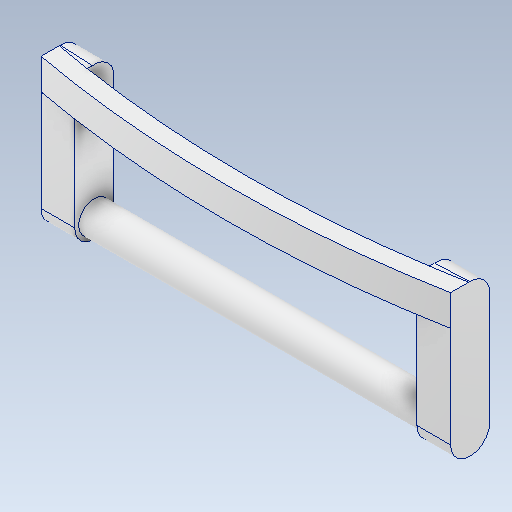
# Autodesk Inventor part: Watch Top strap attachment
Saved by Autodesk Inventor 2020 (Build 240168000, 168)
## iProperties
Created: 2020-05-09
Part Number: Watch Top strap attachment
Material: Aluminum 6061
Document SubType Name: Modeling
Designer: harry
Density: 2.7 g/cm^3
Appearance: Aluminum - Flat
Author: harry
Autodesk Inventor part; units mm, degrees
ref_plane "YZ Plane" through (0, 0, 0) normal (1, 0, 0) x (0, 1, 0)
ref_plane "XY Plane" through (0, 0, 0) normal (0, 0, 1) x (1, 0, 0)
sketch "Sketch1" plane through (0, 0, 0) normal (1, 0, 0) x (0, 1, 0)
  circle A0 centre (0, 0) radius 1.4
  dimension "d0" = 2.8
  constraints: 1 centre point, 1 coincident
  measures "d0" diameter of A0
extrude "Extrusion1" add sketch "Sketch1" along normal mid plane 30.5
sketch "Sketch2" plane through (15.25, 0, 0) normal (1, 0, 0) x (0, 0, -1)
  arc A0 (-1.75, 0) -> (1.75, 0) centre (0, 0) ccw
  line L0 (-1.75, 0) -> (-1.75, 10)
  line L1 (1.75, 0) -> (1.75, 10)
  arc A1 (1.75, 10) -> (-1.75, 10) centre (0, 10) ccw
  dimension "d23" = 1.75
  dimension "d24" = 10
  dimension "d25" = 1.75
  constraints: 4 end point, 4 point on circle, 4 tangent, 2 centre point, 1 coincident, 1 vertical alignment
  measures "d23" radius of A1
  measures "d24" distance of point (0, 0) A1.centre
  measures "d25" radius of A0
extrude "Extrusion2" add sketch "Sketch2" along normal blind 3
mirror "Mirror1" about plane through (0, 0, 0) normal (1, 0, 0) of "Extrusion2"
ref_plane "Work Plane1" through (0, 9, 0) normal (0, 1, 0) x (-1, 0, 0)
sketch "Sketch5" plane through (0, 9, 0) normal (0, 1, 0) x (-1, 0, 0)
  line L0 (18.25, 1.75) -> (18.25, -1.75) projected
  line L1 (-18.25, 1.75) -> (-18.25, -1.75) projected
  arc A0 (18.25, 1.75) -> (-18.25, 1.75) centre (0, -96.5706) ccw
  arc A1 (18.25, 0.1222) -> (-18.25, 0.1222) centre (0, -96.5706) ccw
  line L2 (-18.25, 1.75) -> (-18.25, -1.75) projected
  point P0 (0, 0)
  point P1 (18.25, 0)
  point P2 (-18.25, 0)
  point P3 (-18.25, 0.1222)
  dimension "d26" = 100
  dimension "d27" = 1.6
  constraints: 4 point on circle, 2 centre point, 2 midpoint, 2 vertical alignment
  measures "d26" radius of A0
  measures "d27" radial gap between concentric circles of A0 A1
extrude "Extrusion3" add sketch "Sketch5" along normal blind 2.75
fillet "Fillet1" radius 2 1 edges at (16.7505, 11.7052, 0.3932)
fillet "Fillet2" radius 2 1 edges at (-16.7505, 11.7052, 0.3932)
body "Solid1"
